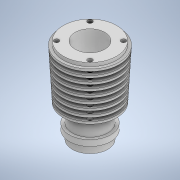
# Autodesk Inventor part: Część24
Saved by Autodesk Inventor 2021 (Build 250183000, 183)
## iProperties
Created: 2023-11-02
Part Number: Część24
Material: Ogólny
Document SubType Name: Modeling
Designer: Jakub
Density: 1 g/cm^3
Appearance: Domyślna
Author: Jakub
Autodesk Inventor part; units mm, degrees
ref_plane "YZ Plane" through (0, 0, 0) normal (1, 0, 0) x (0, 1, 0)
ref_plane "XZ Plane" through (0, 0, 0) normal (0, 1, 0) x (-1, 0, 0)
ref_plane "XY Plane" through (0, 0, 0) normal (0, 0, 1) x (1, 0, 0)
sketch "Szkic2" plane through (0, 0, 0) normal (0, 0, 1) x (1, 0, 0)
  line L0 (0, 0) -> (0, 72)
  line L1 (0, 72) -> (0, 27)
  line L2 (0, 27) -> (62.1065, 27)
  line L3 (0, 72) -> (25, 72)
  line L4 (0, 72) -> (22.5, 72)
  line L5 (22.5, 72) -> (22.5, 69)
  line L6 (25, 72) -> (22.6416, 27)
  line L7 (25, 72) -> (70.0618, 72) construction
  line L8 (22.5, 69) -> (24.8428, 69)
  line L9 (22.5, 69) -> (0, 69)
  line L10 (22.5, 69) -> (22.5, 67)
  line L11 (22.5, 67) -> (24.738, 67)
  line L12 (0, 67) -> (22.5, 67)
  line L13 (22.5, 67) -> (22.5, 64)
  line L14 (22.5, 64) -> (24.5807, 64)
  line L15 (22.5, 64) -> (0, 64)
  line L16 (22.5, 64) -> (22.5, 62)
  line L17 (22.5, 62) -> (24.4759, 62)
  line L18 (22.5, 62) -> (0, 62)
  line L19 (22.5, 62) -> (22.5, 59)
  line L20 (22.5, 59) -> (24.3187, 59)
  line L21 (22.5, 59) -> (0, 59)
  line L22 (22.5, 59) -> (22.5, 57)
  line L23 (22.5, 57) -> (0, 57)
  line L24 (22.5, 57) -> (24.2139, 57)
  line L25 (22.5, 57) -> (22.5, 54)
  line L26 (22.5, 54) -> (0, 54)
  line L27 (22.5, 54) -> (22.5, 52)
  line L28 (22.5, 52) -> (0, 52)
  line L29 (22.5, 52) -> (22.5, 49)
  line L30 (22.5, 49) -> (0, 49)
  line L31 (22.5, 49) -> (22.5, 47)
  line L32 (22.5, 47) -> (0, 47)
  line L33 (22.5, 47) -> (22.5, 44)
  line L34 (22.5, 44) -> (0, 44)
  line L35 (22.5, 44) -> (22.5, 42)
  line L36 (22.5, 42) -> (0, 42)
  line L37 (22.5, 42) -> (22.5, 39)
  line L38 (22.5, 39) -> (0, 39)
  line L39 (22.5, 39) -> (22.5, 37)
  line L40 (22.5, 37) -> (0, 37)
  line L41 (22.5, 37) -> (22.5, 34)
  line L42 (22.5, 34) -> (0, 34)
  line L43 (22.5, 34) -> (22.5, 32)
  line L44 (22.5, 32) -> (0, 32)
  line L45 (22.5, 32) -> (22.5, 29)
  line L46 (22.5, 29) -> (0, 29)
  line L47 (22.5, 29) -> (22.5, 27)
  line L48 (22.5, 29) -> (22.7465, 29)
  line L49 (22.5, 32) -> (22.9037, 32)
  line L50 (22.5, 34) -> (23.0085, 34)
  line L51 (22.5, 37) -> (23.1657, 37)
  line L52 (22.5, 39) -> (23.2705, 39)
  line L53 (22.5, 42) -> (23.4278, 42)
  line L54 (22.5, 44) -> (23.5326, 44)
  line L55 (22.5, 47) -> (23.6898, 47)
  line L56 (22.5, 49) -> (23.7946, 49)
  line L57 (22.5, 52) -> (23.9518, 52)
  line L58 (22.5, 54) -> (24.0567, 54)
  line L59 (0, 27) -> (20, 27)
  line L60 (0, 27) -> (12.5, 27)
  line L61 (0, -14.4) -> (0, 86.4) projected
  line L62 (0, 27) -> (0, 12)
  line L63 (0, 0) -> (0, 5)
  line L64 (18, 27) -> (17, 27)
  line L65 (0, 72) -> (17, 72)
  line L66 (17, 72) -> (17, 27)
  line L67 (0, 27) -> (15, 27)
  line L68 (15, 27) -> (15, 0)
  line L69 (15, 27) -> (15, 12)
  line L70 (15, 12) -> (17.5, 12)
  line L71 (17.5, 12) -> (17.5, 7)
  line L72 (17.5, 7) -> (15, 7)
  line L73 (15, 0) -> (0, 0)
  point P0 (17, 0)
  point P1 (17, 49)
  point P2 (17, 52)
  point P3 (17, 54)
  point P4 (17, 57)
  point P5 (17, 59)
  point P6 (17, 62)
  point P7 (17, 64)
  point P8 (17, 67)
  point P9 (17, 44)
  point P10 (17, 47)
  point P11 (17, 39)
  point P12 (17, 42)
  point P13 (17, 29)
  point P14 (17, 32)
  point P15 (17, 34)
  point P16 (17, 37)
  dimension "d0" = 72
  dimension "d1" = 45
  dimension "d2" = 25
  dimension "d3" = 22.5
  dimension "d4" = 3
  dimension "d5" = 93
  dimension "d6" = 2
  dimension "d7" = 3
  dimension "d8" = 2
  dimension "d9" = 3
  dimension "d10" = 2
  dimension "d11" = 3
  dimension "d12" = 2
  dimension "d13" = 3
  dimension "d14" = 2
  dimension "d15" = 3
  dimension "d16" = 2
  dimension "d17" = 3
  dimension "d18" = 2
  dimension "d19" = 3
  dimension "d20" = 2
  dimension "d21" = 3
  dimension "d22" = 20
  dimension "d24" = 12.5
  dimension "d33" = 15
  dimension "d34" = 5
  dimension "d36" = 1
  dimension "d53" = 15
  dimension "d54" = 15
  dimension "d55" = 2.5
  dimension "d56" = 5
  constraints: 142 end point, 28 point on line, 19 perpendicular, 12 horizontal, 9 parallel, 9 vertical, 40 other
  measures "d0" distance of L0.start L0.end
  measures "d1" distance of L0.end L2.start
  measures "d2" distance of L0.end L3.end
  measures "d3" distance of L0.end L4.end
  measures "d4" distance of L4.end L5.end
  measures "d6" distance of L5.end L10.end
  measures "d7" distance of L10.end L13.end
  measures "d8" distance of L13.end L16.end
  measures "d9" distance of L16.end L19.end
  measures "d10" distance of L19.end L22.end
  measures "d11" distance of L22.end L25.end
  measures "d12" distance of L25.end L27.end
  measures "d13" distance of L27.end L29.end
  measures "d14" distance of L29.end L31.end
  measures "d15" distance of L31.end L33.end
  measures "d16" distance of L33.end L35.end
  measures "d17" distance of L35.end L37.end
  measures "d18" distance of L37.end L39.end
  measures "d19" distance of L39.end L41.end
  measures "d20" distance of L41.end L43.end
  measures "d21" distance of L43.end L45.end
  measures "d22" distance of L2.start L59.end
  measures "d24" distance of L2.start L60.end
  measures "d33" distance of L2.start L62.end
  measures "d34" distance of L0.start L63.end
  measures "d36" distance of L64.start L64.end
  measures "d53" distance of L2.start L67.end
  measures "d54" distance of L67.end L69.end
  measures "d55" distance of L69.end L70.end
  measures "d56" distance of L70.end L71.end
revolve "Obrót1" add sketch "Szkic2" angle 360 about axis through (0, -10, 0) along (0, 1, 0) contours L0 L2 L68 L73 | L68 L70 L71 L72 | L0 L46 L66 L2 | L0 L44 L66 L46 | L0 L42 L66 L44 | L46 L47 L2 L66 | L0 L40 L66 L42 | L66 L42 L43 L44 | L48 L6 L2 L47 | L0 L38 L66 L40 | L43 L50 L6 L49 | L0 L36 L66 L38 | L66 L38 L39 L40 | L0 L34 L66 L36 | L39 L52 L6 L51 | L0 L32 L66 L34 | L66 L34 L35 L36 | L0 L30 L66 L32 | L35 L54 L6 L53 | L0 L28 L66 L30 | L66 L30 L31 L32 | L0 L26 L66 L28 | L31 L56 L6 L55 | L0 L23 L66 L26 | L66 L26 L27 L28 | L0 L21 L66 L23 | L27 L58 L6 L57 | L0 L18 L66 L21 | L66 L21 L22 L23 | L0 L15 L66 L18 | L22 L20 L6 L24 | L0 L12 L66 L15 | L66 L15 L16 L18 | L0 L9 L66 L12 | L16 L14 L6 L17 | L0 L3 L66 L9 | L66 L9 L10 L12 | L66 L3 L5 L9 | L10 L8 L6 L11
sketch "Szkic6" plane through (0, 72, 0) normal (0, 1, 0) x (1, 0, 0)
  circle A0 centre (0, 0) radius 20
  line L0 (0, 0) -> (-14.1421, 14.1421)
  line L1 (0, 0) -> (20, 0) construction
  line L2 (-14.1421, 14.1421) -> (0, 0)
  circle A1 centre (0, 0) radius 22.5 projected
  line L3 (14.1421, -14.1421) -> (0, 0)
  line L4 (0, 0) -> (14.1421, 14.1421)
  line L5 (0, 0) -> (20, 0) construction
  line L6 (14.1421, 14.1421) -> (-14.1421, -14.1421)
  circle A2 centre (-14.1421, -14.1421) radius 2
  circle A3 centre (14.1421, -14.1421) radius 2
  circle A4 centre (14.1421, 14.1421) radius 2
  circle A5 centre (-14.1421, 14.1421) radius 2
  dimension "d57" = 40
  dimension "d58" = 135
  dimension "d59" = 45
  dimension "d60" = 4
  dimension "d61" = 4
  dimension "d62" = 4
  dimension "d63" = 4
  constraints: 14 end point, 5 centre point, 5 coincident, 4 point on circle, 2 collinear, 2 equal length, 2 horizontal, 2 point on line
  measures "d57" diameter of A0
  measures "d58" angle of L1 L0
  measures "d59" angle of L5 L4
  measures "d60" diameter of A2
  measures "d61" diameter of A3
  measures "d62" diameter of A4
  measures "d63" diameter of A5
extrude "Wyciągnięcie proste4" cut sketch "Szkic6" against normal blind 45 contours A4 L4 A0 | A0 A4 | A3 A0 | A0 L3 A3 | L4 A4 A0 | A0 A3 L3 | A5 L0 A0 | A0 A5 | A5 A0 L0 | A2 A0 L6 | L6 A0 A2 | A2 A0
fillet "Zaokrąglenie3" radius 1.5 16 edges at (-17, 42, 0) (-17, 44, 0) (-17, 47, 0) (-17, 67, 0) (-17, 64, 0) (-17, 62, 0) (-17, 59, 0) (-17, 57, 0) (-17, 54, 0) (-17, 52, 0) (-17, 49, 0) (-17, 39, 0) (-17, 37, 0) (-17, 34, 0) (-17, 32, 0) (-17, 29, 0)
sketch "Szkic7" plane through (0, 72, 0) normal (0, 1, 0) x (1, 0, 0)
  circle A0 centre (0, 0) radius 12.5
  dimension "d67" = 25
  constraints: 1 centre point, 1 coincident
  measures "d67" diameter of A0
extrude "Wyciągnięcie proste5" cut sketch "Szkic7" against normal blind 72
chamfer "Faza2" distance 0.5 angle 45 1 edges at (-12.5, 0, 0)
